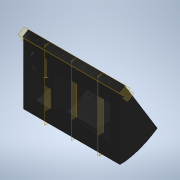
# Autodesk Inventor part: iPadHolder
Saved by Autodesk Inventor 2021.3 (Build 253353000, 353)
## iProperties
Created: 2020-11-06
Part Number: iPadHolder
Material: ポリカーボネート、クリア
Document SubType Name: Modeling
Designer: gisen
Density: 1.2 g/cm^3
Appearance: 滑らか - 黒
Author: gisen
Autodesk Inventor part; units mm, degrees
ref_plane "YZ Plane" through (0, 0, 0) normal (1, 0, 0) x (0, 1, 0)
ref_plane "XZ Plane" through (0, 0, 0) normal (0, 1, 0) x (-1, 0, 0)
ref_plane "XY Plane" through (0, 0, 0) normal (0, 0, 1) x (1, 0, 0)
sketch "スケッチ1" plane through (0, 0, 0) normal (0, 0, 1) x (1, 0, 0)
  line L0 (-116.8004, 49.1733) -> (173.1996, 49.1733)
  line L1 (173.1996, 49.1733) -> (173.1996, -140.8267)
  line L2 (173.1996, -140.8267) -> (-116.8004, -140.8267)
  line L3 (-116.8004, -140.8267) -> (-116.8004, 49.1733)
  point P0 (0, 0)
  dimension "d0" = 290
  dimension "d1" = 190
  constraints: 8 end point, 2 parallel, 1 horizontal, 1 perpendicular
  measures "d0" distance of L0.start L0.end
  measures "d1" distance of L0.end L1.end
extrude "押し出し1" add sketch "スケッチ1" along normal blind 15
sketch "スケッチ2" plane through (0, 0, 15) normal (0, 0, 1) x (1, 0, 0)
  line L0 (163.1996, -133.8267) -> (-95.3004, -133.8267)
  line L1 (-95.3004, -133.8267) -> (-95.3004, 42.1733)
  line L2 (-116.8004, 49.1733) -> (-116.8004, -140.8267) projected
  line L3 (-116.8004, -140.8267) -> (173.1996, -140.8267) projected
  line L4 (173.1996, 49.1733) -> (-116.8004, 49.1733) projected
  line L5 (28.1996, -45.8267) -> (-116.8004, -45.8267)
  line L6 (28.1996, -45.8267) -> (28.1996, 49.1733)
  line L7 (158.1996, 27.1733) -> (158.1996, 42.1733)
  line L8 (158.1996, 27.1733) -> (158.1996, 27.1733)
  line L9 (157.6996, 27.1733) -> (157.6996, 42.1733)
  line L10 (158.1996, -118.8267) -> (158.1996, -118.8267)
  line L11 (157.6996, -118.8267) -> (157.6996, -133.8267)
  line L12 (173.1996, -140.8267) -> (173.1996, 49.1733) projected
  line L13 (157.6996, 42.1733) -> (157.6996, -133.8267)
  line L14 (157.6996, 42.1733) -> (-95.3004, 42.1733)
  point P0 (0, 0)
  dimension "d7" = 7
  dimension "d100" = 15.5
  dimension "d101" = 7
  dimension "d102" = 253
  constraints: 22 end point, 2 midpoint, 2 point on line, 1 collinear, 1 horizontal, 1 perpendicular
  measures "d7" distance between parallel lines of L3 L0
  measures "d100" distance from line of L12 L9.end
  measures "d101" distance from line of L4 L7.end
  measures "d102" distance of L9.end L1.end
ref_plane "作業平面1" through (28.1996, -140.8267, 0) normal (-1, 0, 0) x (0, 0, 1)
ref_plane "作業平面2" through (-116.8004, -45.8267, 0) normal (0, 1, 0) x (1, 0, 0)
extrude "押し出し2" [suppressed]
sketch "スケッチ4" plane through (0, 0, 15) normal (0, 0, 1) x (1, 0, 0)
  circle A0 centre (-106.8004, 39.1733) radius 2.25 projected
  circle A1 centre (163.1996, 39.1733) radius 2.25 projected
  circle A2 centre (163.1996, -130.8267) radius 2.25 projected
  line L0 (173.1996, -140.8267) -> (173.1996, 49.1733) projected
  line L1 (173.1996, 49.1733) -> (-116.8004, 49.1733) projected
  line L2 (-116.8004, 49.1733) -> (-116.8004, -140.8267) projected
  line L3 (-116.8004, -140.8267) -> (173.1996, -140.8267) projected
  circle A3 centre (-106.8004, -130.8267) radius 2.25 projected
  point P0 (0, 0)
hole "穴1" at (-106.8004, 39.1733, 15) at (-106.8004, -130.8267, 15) at (163.1996, -130.8267, 15) at (163.1996, 39.1733, 15) direction (0, 0, -1) diameter 4.5 end through all
ref_plane "作業平面3" through (28.1996, -140.8267, 0) normal (1, 0, 0) x (0, 0, -1)
ref_plane "作業平面4" through (108.1996, -140.8267, 0) normal (1, 0, 0) x (0, 0, -1)
ref_plane "作業平面5" through (-51.8004, -140.8267, 0) normal (1, 0, 0) x (0, 0, -1)
ref_plane "作業平面6" through (108.1996, -140.8267, 0) normal (1, 0, 0) x (0, 0, -1)
sketch "スケッチ6" plane through (108.1996, -140.8267, 0) normal (1, 0, 0) x (0, 0, -1)
  line L0 (-7, 22) -> (-7, 183) projected
  line L1 (0, 190) -> (-15, 190) projected
  line L2 (0, 190) -> (0, 0) projected
  line L3 (-15, 190) -> (-15, 0) projected
  line L4 (0, 0) -> (-15, 0) projected
  line L5 (-15, 190) -> (-18, 190)
  line L6 (-18, 190) -> (-0.9497, 200.4541)
  line L7 (-0.9497, 200.4541) -> (98.3645, 38.4767)
  line L8 (98.3645, 38.4767) -> (81.3143, 28.0226)
  arc A0 (0, 0) -> (81.3143, 28.0226) centre (-28.8813, 215.7937) ccw
  point P0 (-7, 7)
  dimension "d51" = 3
  dimension "d52" = 20
  dimension "d53" = 190
  dimension "d54" = 20
  constraints: 8 end point, 2 perpendicular, 2 point on circle, 1 centre point, 1 horizontal
  measures "d51" distance of L1.end L5.end
  measures "d52" distance of L5.end L6.end
  measures "d53" distance of L6.end L7.end
  measures "d54" distance of L7.end L8.end
extrude "押し出し5" add sketch "スケッチ6" against normal blind 20 contours L1 L5 L6 L7 L8 A0 L2
sketch "スケッチ8" plane through (173.1996, -140.8267, 0) normal (1, 0, 0) x (0, 0, -1)
  line L0 (81.3143, 28.0226) -> (98.3645, 38.4767) projected
  line L1 (98.3645, 38.4767) -> (-0.9497, 200.4541) projected
  line L2 (-0.9497, 200.4541) -> (-18, 190) projected
  line L3 (-18, 190) -> (-15, 190) projected
  line L4 (0, 190) -> (-15, 190) projected
  line L5 (0, 0) -> (0, 190) projected
  arc A0 (0, 0) -> (81.3143, 28.0226) centre (-28.8813, 215.7937) ccw projected
  line L6 (98.3645, 38.4767) -> (-0.9497, 200.4541) projected
  line L7 (95.751, 42.7393) -> (78.7007, 32.2852)
  line L8 (0, 0) -> (0, 190) projected
  line L9 (4.2773, 191.929) -> (0, 189.3064)
  arc A1 (0, 5.0447) -> (78.7007, 32.2852) centre (-28.8813, 215.7937) ccw
  point P0 (0, 140.8267)
  point P1 (95.751, 42.7393)
  dimension "d57" = 20
  dimension "d58" = 5
  dimension "d60" = 10
  constraints: 4 end point, 4 point on line, 2 parallel, 2 point on circle, 1 centre point, 1 concentric, 1 perpendicular
  measures "d57" distance of L7.start L7.end
  measures "d58" distance of L0.end L7.start
  measures "d60" distance of L1.end L9.start
extrude "押し出し6" add sketch "スケッチ8" against normal up to surface (290 mm away) contours A0 L5 A1 L7 L1 L0 | L9 L5 L4 L3 L2 L1
sketch "スケッチ9" plane through (173.1996, -140.8267, 15) normal (1, 0, 0) x (0, 0, -1)
  line L0 (15, 5.0447) -> (15, 189.3064) projected
  line L1 (15, 189.3064) -> (19.2773, 191.929) projected
  line L2 (19.2773, 191.929) -> (14.0503, 200.4541) projected
  line L3 (14.0503, 200.4541) -> (-3, 190) projected
  line L4 (-3, 190) -> (0, 190) projected
  line L5 (0, 0) -> (0, 190) projected
  line L6 (15, 0) -> (0, 0) projected
  arc A0 (15, 0) -> (96.3143, 28.0226) centre (-13.8813, 215.7937) ccw projected
  line L7 (96.3143, 28.0226) -> (113.3645, 38.4767) projected
  line L8 (113.3645, 38.4767) -> (110.751, 42.7393) projected
  line L9 (110.751, 42.7393) -> (93.7007, 32.2852) projected
  arc A1 (15, 5.0447) -> (93.7007, 32.2852) centre (-13.8813, 215.7937) ccw projected
  arc A2 (15, 5.0447) -> (93.7007, 32.2852) centre (-13.8813, 215.7937) ccw projected
  line L10 (93.7007, 32.2852) -> (110.751, 42.7393) projected
  line L11 (110.751, 42.7393) -> (19.2773, 191.929) projected
  line L12 (19.2773, 191.929) -> (15, 189.3064) projected
  line L13 (15, 5.0447) -> (15, 189.3064) projected
  point P0 (15, 140.8267)
extrude "押し出し7" add sketch "スケッチ9" against normal blind 5 contours L0 L1 L11 L9 A1
mirror "ミラー3" about plane through (28.1996, -140.8267, 0) normal (1, 0, 0) of "押し出し5", "押し出し7"
sketch "スケッチ10" plane through (-31.8004, -108.5415, -78.7007) normal (0, 0.8525126, 0.5227067) x (1, 0, 0)
  line L0 (0, 20) -> (0, 0) projected
  line L1 (120, 0) -> (0, 0) projected
  line L2 (120, 20) -> (120, 0) projected
  line L3 (120, 20) -> (0, 20) projected
  line L4 (200, 20) -> (140, 20) projected
  line L5 (60, 145.4629) -> (60, -140.1105) projected
  line L6 (140, 0) -> (140, 20) projected
  point P0 (31.8004, -10.358)
  point P1 (90, 10)
  point P2 (170, 10)
  point P3 (30, 10)
  point P4 (-50, 10)
  dimension "d66" = 10
  dimension "d67" = 10
  dimension "d68" = 30
  dimension "d69" = 30
  constraints: 2 symmetric about line
  measures "d66" distance from line of L4 point (170, 10)
  measures "d67" distance from line of L3 point (90, 10)
  measures "d68" distance from line of L5 point (90, 10)
  measures "d69" distance from line of L6 point (170, 10)
hole "穴3" at (58.1996, -103.3144, -87.2259) at (138.1996, -103.3144, -87.2259) at (-81.8004, -103.3144, -87.2259) at (-1.8004, -103.3144, -87.2259) direction (0, -0.8525126, -0.5227067) diameter 4.5 end through all
sketch "スケッチ11" plane through (-31.8004, 59.6275, 0.9497) normal (0, -0.8525126, -0.5227067) x (1, 0, 0)
  circle A0 centre (30, 10) radius 2.25 projected
  circle A1 centre (90, 10) radius 2.25 projected
  circle A2 centre (-50, 10) radius 2.25 projected
  circle A3 centre (170, 10) radius 2.25 projected
  point P0 (31.8004, 30.358)
hole "穴4" at (-81.8004, 54.4004, 9.4749) at (-1.8004, 54.4004, 9.4749) at (58.1996, 54.4004, 9.4749) at (138.1996, 54.4004, 9.4749) direction (0, -0.8525126, -0.5227067) diameter 4.5 end through all
ref_plane "作業平面8" through (-116.8004, 46.6158, 16.4319) normal (0, 0.8525126, 0.5227067) x (1, 0, 0)
ref_plane "作業平面11" through (-116.8004, 27.8605, 4.9323) normal (0, 0.8525126, 0.5227067) x (1, 0, 0)
sketch "スケッチ14" plane through (-116.8004, 27.8605, 4.9323) normal (0, 0.8525126, 0.5227067) x (1, 0, 0)
  circle A0 centre (115, 10) radius 2.25 projected
  circle A1 centre (175, 10) radius 2.25 projected
  circle A2 centre (255, 10) radius 2.25 projected
  circle A3 centre (35, 10) radius 2.25 projected
  point P0 (116.8004, -10.358)
hole "穴6" at (-81.8004, 33.0876, -3.5928) at (-1.8004, 33.0876, -3.5928) at (58.1996, 33.0876, -3.5928) at (138.1996, 33.0876, -3.5928) direction (0, 0.8525126, 0.5227067) diameter 8 depth 22
ref_plane "作業平面12" through (-95.3004, -45.8267, 15) normal (0, -1, 0) x (1, 0, 0)
sketch "スケッチ15" plane through (0, 0, 15) normal (0, 0, 1) x (1, 0, 0)
  circle A0 centre (163.1996, -130.8267) radius 2.25 projected
  circle A1 centre (-106.8004, 39.1733) radius 2.25 projected
  circle A2 centre (-106.8004, -130.8267) radius 2.25 projected
  circle A3 centre (163.1996, 39.1733) radius 2.25 projected
  line L0 (-116.8004, -140.8267) -> (173.1996, -140.8267) projected
  line L1 (173.1996, -140.8267) -> (173.1996, 49.1733) projected
  line L2 (173.1996, 49.1733) -> (-116.8004, 49.1733) projected
  line L3 (-116.8004, 49.1733) -> (-116.8004, -140.8267) projected
  line L4 (231.1996, -45.8267) -> (-174.8004, -45.8267) projected
  line L5 (-95.3004, -54.3995) -> (-95.3004, -37.2538) construction
  line L6 (-95.3004, -133.8267) -> (-95.3004, 42.1733) projected
  line L7 (-85.3004, -54.3995) -> (-85.3004, -37.2538)
  line L8 (-105.3004, -37.2538) -> (-105.3004, -54.3995)
  arc A4 (-105.3004, -54.3995) -> (-85.3004, -54.3995) centre (-95.3004, -54.3995) ccw
  arc A5 (-85.3004, -37.2538) -> (-105.3004, -37.2538) centre (-95.3004, -37.2538) ccw
  line L9 (-95.3004, -133.8267) -> (-95.3004, 42.1733) projected
  point P0 (0, 0)
  point P1 (-95.3004, -45.8267)
  point P2 (-85.3004, -45.8267)
  point P3 (173.1996, -45.8267)
  point P4 (-116.8004, -45.8267)
  point P5 (-105.3004, -45.8267)
  dimension "d103" = 20
  constraints: 8 end point, 4 point on circle, 4 tangent, 2 centre point, 2 midpoint, 1 parallel, 1 point on line
  measures "d103" distance between parallel lines of L7 L8
extrude "押し出し8" [suppressed]
sketch "スケッチ17" plane through (-116.8004, -140.8267, 15) normal (-1, 0, 0) x (0, 0, 1)
  line L0 (-15, 0) -> (0, 0) projected
  line L1 (0, 190) -> (0, 0) projected
  line L2 (-113.3645, 38.4767) -> (-14.0503, 200.4541) projected
  line L3 (-96.3143, 28.0226) -> (-113.3645, 38.4767) projected
  arc A0 (-96.3143, 28.0226) -> (-15, 0) centre (13.8813, 215.7937) ccw projected
  line L4 (3, 190) -> (0, 190) projected
  line L5 (-14.0503, 200.4541) -> (3, 190) projected
  point P0 (-15, 140.8267)
  point P1 (-78.7041, 75.8753)
  point P2 (-36.8875, 144.0763)
hole "穴7" at (-116.8004, 3.2496, -21.8875) at (-116.8004, -64.9514, -63.7041) direction (1, 0, 0) diameter 4.5 depth 5
mirror "ミラー4" about plane through (28.1996, -140.8267, 0) normal (1, 0, 0) of "穴7"
sketch "スケッチ18" plane through (0, 0, 15) normal (0, 0, 1) x (1, 0, 0)
  line L0 (-36.3004, -48.3267) -> (-97.3004, -48.3267)
  line L1 (-99.3004, -50.3267) -> (-99.3004, -111.3267)
  line L2 (-34.3004, -111.3267) -> (-34.3004, -50.3267)
  line L3 (-97.3004, -113.3267) -> (-36.3004, -113.3267)
  line L4 (-100.3004, -47.3267) -> (-33.3004, -47.3267)
  line L5 (-33.3004, -47.3267) -> (-33.3004, -114.3267)
  line L6 (-33.3004, -114.3267) -> (-100.3004, -114.3267)
  line L7 (-100.3004, -114.3267) -> (-100.3004, -47.3267)
  point P0 (0, 0)
  dimension "d117" = 1
  dimension "d118" = 1
  dimension "d119" = 1
  dimension "d120" = 1
  constraints: 16 end point, 3 horizontal, 2 parallel, 2 vertical, 1 perpendicular, 8 other
  measures "d117" distance between parallel lines of L4 L0
  measures "d118" distance between parallel lines of L6 L3
  measures "d119" distance between parallel lines of L7 L1
  measures "d120" distance between parallel lines of L5 L2
extrude "押し出し9" cut sketch "スケッチ18" against normal blind 20
sketch "スケッチ19" plane through (0, 0, 15) normal (0, 0, 1) x (1, 0, 0)
  line L0 (-23.6004, -95.9767) -> (143.1996, -95.9767)
  line L1 (-23.6004, 4.3233) -> (-23.6004, -95.9767)
  line L2 (143.1996, 4.3233) -> (-23.6004, 4.3233)
  line L3 (143.1996, -95.9767) -> (143.1996, 4.3233)
  line L4 (-24.6004, 5.3233) -> (144.1996, 5.3233)
  line L5 (144.1996, 5.3233) -> (144.1996, -96.9767)
  line L6 (144.1996, -96.9767) -> (-24.6004, -96.9767)
  line L7 (-24.6004, -96.9767) -> (-24.6004, 5.3233)
  point P0 (0, 0)
  dimension "d123" = 1
  dimension "d124" = 1
  dimension "d125" = 1
  dimension "d126" = 1
  constraints: 16 end point, 3 horizontal, 2 parallel, 2 vertical, 1 perpendicular, 4 other
  measures "d123" distance between parallel lines of L7 L1
  measures "d124" distance between parallel lines of L4 L2
  measures "d125" distance between parallel lines of L3 L5
  measures "d126" distance between parallel lines of L6 L0
extrude "押し出し10" cut sketch "スケッチ19" against normal through all contours L1 L2 L3 L0 | L4 L5 L6 L7
sketch "スケッチ20" plane through (0, 0, 15) normal (0, 0, 1) x (1, 0, 0)
  circle A0 centre (-66.8004, -0.8267) radius 29.75
  circle A1 centre (-66.8004, -0.8267) radius 30.75
  point P0 (0, 0)
  dimension "d129" = 1
  constraints: 2 centre point, 1 coincident, 2 other
  measures "d129" radial gap between concentric circles of A1 A0
extrude "押し出し11" cut sketch "スケッチ20" against normal blind 5.5 contours A0 | A1
sketch "スケッチ21" plane through (0, 0, 15) normal (0, 0, 1) x (1, 0, 0)
  circle A0 centre (-18.7004, 12.0233) radius 1.75
  circle A1 centre (138.2996, 12.0233) radius 1.75
  circle A2 centre (138.2996, -103.6767) radius 1.75
  circle A3 centre (-18.7004, -103.6767) radius 1.75
  point P0 (0, 0)
  constraints: 4 centre point, 8 other
hole "穴8" at (-18.7004, 12.0233, 15) at (-18.7004, -103.6767, 15) at (138.2996, -103.6767, 15) at (138.2996, 12.0233, 15) direction (0, 0, -1) diameter 4.5 end through all
